Autodesk Fusion 360 part; units mm, degrees
(part 2 of 2)
sketch "Sketch7" plane through (0, 0, 200) normal (0, 0, 1) x (1, 0, 0)
  line L0 (5, 10) -> (-5, 10)
  line L1 (-5, 10) -> (-6.8, 8.2)
  line L2 (-6.8, 8.2) -> (-5, 8.2)
  line L3 (-5, 8.2) -> (-5, 6.4)
  line L4 (-5, 6.4) -> (-7.4, 4)
  line L5 (-7.4, 4) -> (-12.6, 4)
  line L6 (-12.6, 4) -> (-15, 6.4)
  line L7 (-15, 6.4) -> (-15, 8.2)
  line L8 (-15, 8.2) -> (-13.2, 8.2)
  line L9 (-13.2, 8.2) -> (-15, 10)
  line L10 (-15, 10) -> (-19.5, 10)
  arc A0 (-19.5, 10) -> (-20, 9.5) centre (-19.5, 9.5) ccw
  line L11 (-20, 9.5) -> (-20, 5)
  line L12 (-20, 5) -> (-18.2, 3.2)
  line L13 (-18.2, 3.2) -> (-18.2, 5)
  line L14 (-18.2, 5) -> (-16.4, 5)
  line L15 (-16.4, 5) -> (-14, 2.6)
  line L16 (-14, 2.6) -> (-14, -2.6)
  line L17 (-14, -2.6) -> (-16.4, -5)
  line L18 (-16.4, -5) -> (-18.2, -5)
  line L19 (-18.2, -5) -> (-18.2, -3.2)
  line L20 (-18.2, -3.2) -> (-20, -5)
  line L21 (-20, -5) -> (-20, -9.5)
  arc A1 (-20, -9.5) -> (-19.5, -10) centre (-19.5, -9.5) ccw
  line L22 (-19.5, -10) -> (-15, -10)
  line L23 (-15, -10) -> (-13.2, -8.2)
  line L24 (-13.2, -8.2) -> (-15, -8.2)
  line L25 (-15, -8.2) -> (-15, -6.4)
  line L26 (-15, -6.4) -> (-12.6, -4)
  line L27 (-12.6, -4) -> (-7.4, -4)
  line L28 (-7.4, -4) -> (-5, -6.4)
  line L29 (-5, -6.4) -> (-5, -8.2)
  line L30 (-5, -8.2) -> (-6.8, -8.2)
  line L31 (-6.8, -8.2) -> (-5, -10)
  line L32 (-5, -10) -> (5, -10)
  line L33 (5, -10) -> (6.8, -8.2)
  line L34 (6.8, -8.2) -> (5, -8.2)
  line L35 (5, -8.2) -> (5, -6.4)
  line L36 (5, -6.4) -> (7.4, -4)
  line L37 (7.4, -4) -> (12.6, -4)
  line L38 (12.6, -4) -> (15, -6.4)
  line L39 (15, -6.4) -> (15, -8.2)
  line L40 (15, -8.2) -> (13.2, -8.2)
  line L41 (13.2, -8.2) -> (15, -10)
  line L42 (15, -10) -> (19.5, -10)
  arc A2 (19.5, -10) -> (20, -9.5) centre (19.5, -9.5) ccw
  line L43 (20, -9.5) -> (20, -5)
  line L44 (20, -5) -> (18.2, -3.2)
  line L45 (18.2, -3.2) -> (18.2, -5)
  line L46 (18.2, -5) -> (16.4, -5)
  line L47 (16.4, -5) -> (14, -2.6)
  line L48 (14, -2.6) -> (14, 2.6)
  line L49 (14, 2.6) -> (16.4, 5)
  line L50 (16.4, 5) -> (18.2, 5)
  line L51 (18.2, 5) -> (18.2, 3.2)
  line L52 (18.2, 3.2) -> (20, 5)
  line L53 (20, 5) -> (20, 9.5)
  arc A3 (20, 9.5) -> (19.5, 10) centre (19.5, 9.5) ccw
  line L54 (19.5, 10) -> (15, 10)
  line L55 (15, 10) -> (13.2, 8.2)
  line L56 (13.2, 8.2) -> (15, 8.2)
  line L57 (15, 8.2) -> (15, 6.4)
  line L58 (15, 6.4) -> (12.6, 4)
  line L59 (12.6, 4) -> (7.4, 4)
  line L60 (7.4, 4) -> (5, 6.4)
  line L61 (5, 6.4) -> (5, 8.2)
  line L62 (5, 8.2) -> (6.8, 8.2)
  line L63 (6.8, 8.2) -> (5, 10)
  circle A4 centre (10, 0) radius 2.5
  line L64 (0, 5) -> (1.8, 3.2)
  line L65 (1.8, 3.2) -> (1.8, 5)
  line L66 (1.8, 5) -> (3.6, 5)
  line L67 (3.6, 5) -> (6, 2.6)
  line L68 (6, 2.6) -> (6, -2.6)
  line L69 (6, -2.6) -> (3.6, -5)
  line L70 (3.6, -5) -> (1.8, -5)
  line L71 (1.8, -5) -> (1.8, -3.2)
  line L72 (1.8, -3.2) -> (0, -5)
  line L73 (0, -5) -> (-1.8, -3.2)
  line L74 (-1.8, -3.2) -> (-1.8, -5)
  line L75 (-1.8, -5) -> (-3.6, -5)
  line L76 (-3.6, -5) -> (-6, -2.6)
  line L77 (-6, -2.6) -> (-6, 2.6)
  line L78 (-6, 2.6) -> (-3.6, 5)
  line L79 (-3.6, 5) -> (-1.8, 5)
  line L80 (-1.8, 5) -> (-1.8, 3.2)
  line L81 (-1.8, 3.2) -> (0, 5)
  circle A5 centre (-10, 0) radius 2.5
  line L82 (-17, -7) -> (-18, -7)
  line L83 (-18, -7) -> (-18, -8)
  line L84 (-18, -8) -> (-17, -8)
  line L85 (-17, -8) -> (-17, -7)
  line L86 (-17, 7) -> (-17, 8)
  line L87 (-17, 8) -> (-18, 8)
  line L88 (-18, 8) -> (-18, 7)
  line L89 (-18, 7) -> (-17, 7)
  line L90 (17, 7) -> (18, 7)
  line L91 (18, 7) -> (18, 8)
  line L92 (18, 8) -> (17, 8)
  line L93 (17, 8) -> (17, 7)
  line L94 (17, -7) -> (17, -8)
  line L95 (17, -8) -> (18, -8)
  line L96 (18, -8) -> (18, -7)
  line L97 (18, -7) -> (17, -7)
  line L98 (3, -8) -> (3, -5.5716)
  line L99 (3, -5.5716) -> (6.5716, -2)
  line L100 (6.5716, -2) -> (12, -2)
  line L101 (12, -2) -> (12, 2)
  line L102 (12, 2) -> (6.5716, 2)
  line L103 (6.5716, 2) -> (3, 5.5716)
  line L104 (3, 5.5716) -> (3, 8)
  line L105 (3, 8) -> (-3, 8)
  line L106 (-3, 8) -> (-3, 5.5716)
  line L107 (-3, 5.5716) -> (-6.5716, 2)
  line L108 (-6.5716, 2) -> (-12, 2)
  line L109 (-12, 2) -> (-12, -2)
  line L110 (-12, -2) -> (-6.5716, -2)
  line L111 (-6.5716, -2) -> (-3, -5.5716)
  line L112 (-3, -5.5716) -> (-3, -8)
  line L113 (-3, -8) -> (3, -8)
  dimension "d51" = -2
extrude "Extrude7" cut sketch "Sketch7" against normal blind 400 contours L64 L65 L66 L79 L80 L81 L103 L104 L105 L106 L107 | L70 L71 L72 L73 L74 L75 L98 L99 L111 L112 L113 bodies 1
equation "d23 = -length / 2"
equation "length = 400 mm"
equation "d52 = -length"
named bodies: "2040", "2060", "2080", "2020", "2020 (1)", "2040 (1)", "2060 (1)", "2080 (1)"
